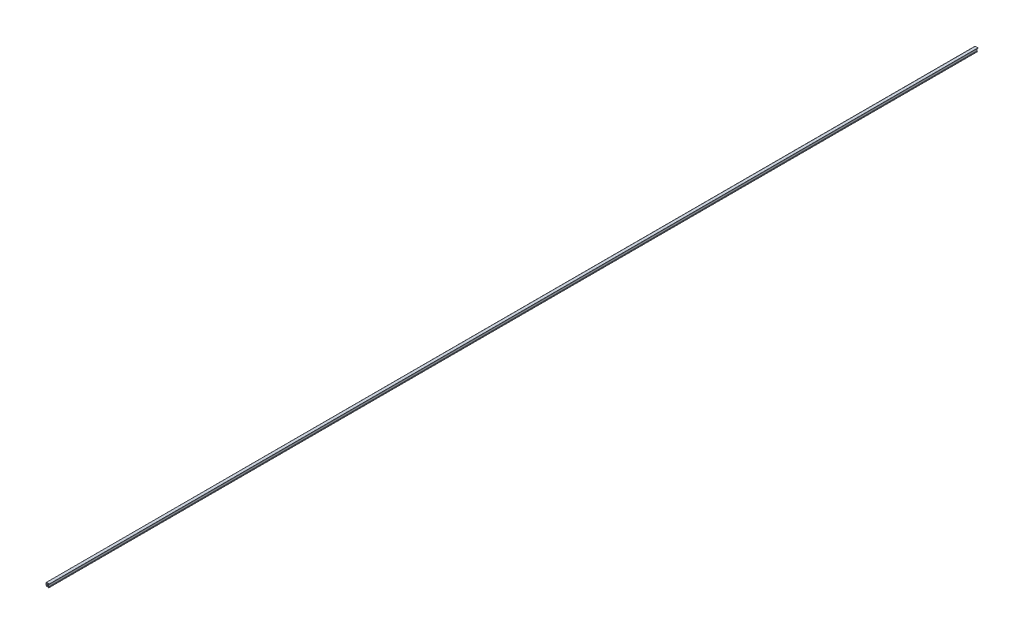
# Autodesk Inventor part: SP40-08 JUNQUILLO CURVO
Saved by Autodesk Inventor 2025 (Build 290162000, 162)
## iProperties
Created: 2026-01-26
Part Number: SP40-08 JUNQUILLO CURVO
Material: Aluminio
Document SubType Name: Modeling
Designer: ROLANDO
Density: 2.7 g/cm^3
Appearance: Satinado
Author: ROLANDO
Autodesk Inventor part; units mm, degrees
ref_plane "YZ Plane" through (0, 0, 0) normal (1, 0, 0) x (0, 1, 0)
ref_plane "XZ Plane" through (0, 0, 0) normal (0, 1, 0) x (-1, 0, 0)
ref_plane "XY Plane" through (0, 0, 0) normal (0, 0, 1) x (1, 0, 0)
sketch "Boceto1" plane through (0, 0, 0) normal (0, 0, 1) x (1, 0, 0)
  line L0 (-1.6474, 10.1749) -> (-1.6474, 19.8749)
  line L1 (-1.1474, 9.6749) -> (1.7348, 9.6749)
  line L2 (0.4348, 8.3749) -> (-2.9474, 8.3749)
  line L3 (0.4348, 8.3749) -> (0.4348, 6.5749)
  line L4 (0.8274, 3.9949) -> (0.9348, 3.9949)
  line L5 (1.7348, 4.7949) -> (1.7348, 9.6749)
  line L6 (-1.6474, 19.8749) -> (-0.7874, 19.8749)
  line L7 (-0.3874, 20.2749) -> (-0.3874, 23.4749)
  line L8 (1.0526, 26.7749) -> (17.5526, 26.7749)
  line L9 (11.7826, 25.4749) -> (11.7826, 6.3904)
  line L10 (10.4826, 6.1804) -> (10.4826, 25.4749)
  line L11 (0.4348, 6.5749) -> (-0.6652, 6.5749)
  line L12 (15.8805, 25.4749) -> (11.7826, 25.4749)
  line L13 (10.4826, 25.4749) -> (1.6126, 25.4749)
  line L14 (18.0526, 26.2749) -> (18.0526, 24.4749)
  line L15 (18.0526, 24.4749) -> (16.7881, 24.4749)
  line L16 (-2.9474, 22.7749) -> (-2.9474, 8.3749)
  line L17 (0.372, 4.2883) -> (-0.6652, 6.5749)
  arc A0 (0.9348, 3.9949) -> (1.7348, 4.7949) centre (0.9348, 4.7949) ccw
  arc A1 (0.372, 4.2883) -> (0.8274, 3.9949) centre (0.8274, 4.4949) ccw
  arc A2 (-1.6474, 10.1749) -> (-1.1474, 9.6749) centre (-1.1474, 10.1749) ccw
  arc A3 (1.0526, 26.7749) -> (-2.9474, 22.7749) centre (1.0526, 22.7749) ccw
  arc A4 (1.6126, 25.4749) -> (-0.3874, 23.4749) centre (1.6126, 23.4749) ccw
  arc A5 (-0.7874, 19.8749) -> (-0.3874, 20.2749) centre (-0.7874, 20.2749) ccw
  line L18 (16.3655, 24.7077) -> (15.8805, 25.4749)
  arc A6 (16.3655, 24.7077) -> (16.7881, 24.4749) centre (16.7881, 24.9749) ccw
  arc A7 (18.0526, 26.2749) -> (17.5526, 26.7749) centre (17.5526, 26.2749) ccw
  line L19 (13.2948, 10.0513) -> (13.2948, 2.2212) construction
  line L20 (10.8004, 4.1149) -> (18.33, 4.1149) construction
  line L21 (16.0504, 5.6012) -> (14.3604, 4.457)
  line L22 (10.8864, 5.3776) -> (12.0584, 4.5072)
  arc A8 (12.0584, 4.5072) -> (14.3604, 4.457) centre (13.2448, 6.1047) ccw
  arc A9 (12.6335, 5.6403) -> (13.7963, 5.5253) centre (13.2948, 6.3904) ccw
  line L23 (11.7826, 6.3904) -> (15.1894, 6.3904) construction
  line L24 (11.7826, 6.3904) -> (12.6335, 5.6403)
  line L25 (15.4813, 6.502) -> (13.7963, 5.5253)
  arc A10 (10.4826, 6.1804) -> (10.8864, 5.3776) centre (11.4826, 6.1804) ccw
  line L26 (16.2648, 6.2046) -> (16.2603, 6.2181)
  arc A11 (16.2648, 6.2046) -> (15.4813, 6.502) centre (15.7522, 6.0349) ccw
  arc A12 (16.0504, 5.6012) -> (16.2603, 6.2181) centre (15.7477, 6.0484) ccw
  point P0 (0, 0)
  point P1 (0.5051, 3.9949)
  point P2 (18.0526, 26.7749)
  point P3 (16.5126, 24.4749)
  point P4 (12.2081, 6.0154)
  point P5 (16.2626, 6.2113)
  point P6 (15.9438, 6.5397)
  point P7 (13.2014, 4.1153)
  point P8 (16.2625, 6.2113)
  dimension "d1" = 22.78
  dimension "d2" = 1.3
  dimension "d3" = 1.3
  dimension "d4" = 1.3
  dimension "d5" = 1.3
  dimension "d6" = 1.3
  dimension "d9" = 1.8
  dimension "d10" = 1.1
  dimension "d14" = 0.8
  dimension "d15" = 0.5
  dimension "d16" = 65.6
  dimension "d17" = 2.3
  dimension "d18" = 18.4
  dimension "d19" = 0.5
  dimension "d21" = 4
  dimension "d23" = 2.56
  dimension "d24" = 21
  dimension "d27" = 2
  dimension "d28" = 14.73
  dimension "d29" = 0.4
  dimension "d30" = 1.54
  dimension "d31" = 57.7
  dimension "d32" = 0.5
  dimension "d33" = 0.5
  dimension "d61" = 34.1
  dimension "d63" = 2
  dimension "d65" = 48.6
  dimension "d66" = 59.9
  dimension "d69" = 0.29
  dimension "d70" = 1
  dimension "d83" = 6.9
  dimension "d84" = 22.66
  dimension "d87" = 36.6
  dimension "d93" = 0.05
  dimension "d95" = 1.3
  dimension "d102" = 0.54
  dimension "d104" = 3.02
  dimension "d107" = 2.46
  dimension "d108" = 15.83
  dimension "d109" = 19.2077
  dimension "d110" = 18.0526
  dimension "d111" = 24.4748
  dimension "d112" = 0.2774
  dimension "d113" = 2.8632
  dimension "d114" = 14.4235
  dimension "d115" = 22.2536
  dimension "d116" = 7.2522
  constraints: 54 end point, 28 point on circle, 27 tangent, 13 centre point, 8 point on line, 6 horizontal, 6 parallel, 4 perpendicular, 3 vertical, 2 midpoint, 1 collinear, 1 equal radius
  measures "d1" distance between parallel lines of L4 L8
  measures "d2" distance between parallel lines of L8 L13
  measures "d3" distance between parallel lines of L1 L2
  measures "d4" distance between parallel lines of L5 L3
  measures "d5" distance between parallel lines of L16 L0
  measures "d6" distance between parallel lines of L10 L9
  measures "d9" distance between parallel lines of L11 L2
  measures "d10" distance of L3.end L11.end
  measures "d14" radius of A0
  measures "d15" radius of A1
  measures "d16" angle of L11 L17
  measures "d17" distance of point (18.053, 26.775) L14.end
  measures "d18" distance between parallel lines of L8 L2
  measures "d19" radius of A2
  measures "d21" radius of A3
  measures "d23" distance between parallel lines of L16 L7
  measures "d24" distance between parallel lines of L14 L16
  measures "d27" radius of A4
  measures "d28" distance between parallel lines of L9 L16
  measures "d29" radius of A5
  measures "d30" distance of L14.end point (16.513, 24.475)
  measures "d31" angle of L15 L18
  measures "d32" radius of A6
  measures "d33" radius of A7
  measures "d61" angle of L21 L20
  measures "d63" diameter of A9
  measures "d65" angle of L24 L19
  measures "d66" angle of L25 L19
  measures "d69" distance of A8.centre A9.centre
  measures "d70" radius of A10
  measures "d83" distance between parallel lines of L8 L6
  measures "d87" angle of L20 L22
  measures "d93" horizontal distance of A9.centre A8.centre
  measures "d95" distance from line of point (12.208, 6.015) L22
  measures "d102" radius of A11
  measures "d104" horizontal distance of L26.start A8.centre
  measures "d108" distance from line of L26.start L3
  measures "d109" distance from line of L26.end L16
  measures "d110" distance from line of point (0, 0) L14
  measures "d111" distance from line of point (0, 0) L15
  measures "d112" distance from line of L20.end L14
  measures "d113" distance from line of L23.end L14
  measures "d114" distance from line of L19.start L15
  measures "d115" distance from line of L19.end L15
  measures "d116" distance from line of L20.start L14
extrude "Extrusión1" add sketch "Boceto1" against normal blind 5800
